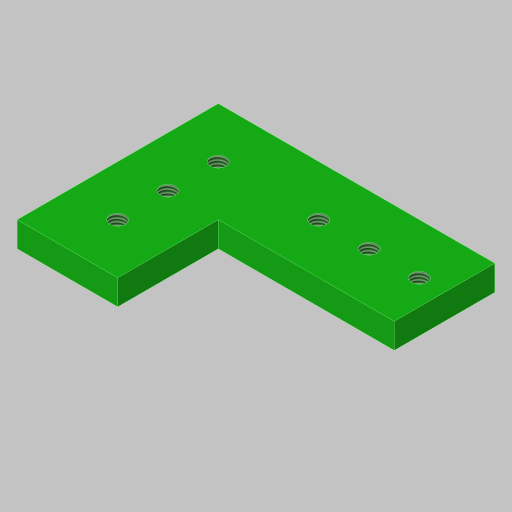
# Autodesk Inventor part: DB1-004
Saved by Autodesk Inventor 2023.5 (Build 275446000, 446)
## iProperties
Created: 2025-01-09
Part Number: DB1-004
Material: Aluminum 6061
Document SubType Name: Modeling
Designer: mavericks
Density: 2.7 g/cm^3
Appearance: Dark Green
Author: mavericks
Autodesk Inventor part; units mm, degrees
ref_plane "YZ Plane" through (0, 0, 0) normal (1, 0, 0) x (0, 1, 0)
ref_plane "XZ Plane" through (0, 0, 0) normal (0, 1, 0) x (-1, 0, 0)
ref_plane "XY Plane" through (0, 0, 0) normal (0, 0, 1) x (1, 0, 0)
sketch "Sketch1" plane through (0, 0, 0) normal (0, 1, 0) x (-1, 0, 0)
  line L0 (12.7, 25.4) -> (-12.7, 25.4)
  line L1 (-12.7, 25.4) -> (-12.7, -25.4)
  line L2 (-12.7, -25.4) -> (12.7, -25.4)
  line L3 (12.7, -25.4) -> (12.7, 25.4)
  line L4 (12.7, 25.4) -> (-12.7, -25.4) construction
  line L5 (-12.7, 25.4) -> (12.7, -25.4) construction
  point P0 (0, 0)
  dimension "d0" = 25.4
  dimension "d1" = 50.8
  constraints: 12 end point, 2 midpoint, 2 parallel, 1 horizontal, 1 perpendicular
  measures "d0" distance of L2.end L1.end
  measures "d1" distance of L1.end L0.end
extrude "Extrusion1" add sketch "Sketch1" along normal blind 6.35
sketch "Sketch3" plane through (12.7, 0, 25.4) normal (1, 0, 0) x (0, 0, -1)
  line L0 (0, 6.35) -> (50.8, 6.35) projected
  line L1 (50.8, 6.35) -> (25.4, 6.35)
  line L2 (25.4, 6.35) -> (25.4, 0)
  line L3 (25.4, 0) -> (50.8, 0)
  line L4 (50.8, 0) -> (50.8, 6.35)
  dimension "d14" = 25.4
  constraints: 8 end point, 2 parallel, 1 horizontal, 1 perpendicular
  measures "d14" distance of L3.end L2.end
extrude "Extrusion2" add sketch "Sketch3" along normal blind 44.45
sketch "Sketch4" plane through (0, 6.35, 0) normal (0, 1, 0) x (1, 0, 0)
  line L0 (-12.7, -25.4) -> (12.7, -25.4) projected
  point P0 (0, 0)
  point P1 (0, -12.7)
  point P2 (0, 0)
  point P3 (0, 12.7)
  point P4 (0, -25.4)
  point P5 (0, -25.4)
  point P6 (0, -25.4)
  point P7 (25.4, 12.7)
  point P8 (38.1, 12.7)
  point P9 (50.8, 12.7)
  dimension "d17" = 12.7
  dimension "d18" = 12.7
  dimension "d19" = 12.7
  dimension "d20" = 25.4
  dimension "d21" = 12.7
  dimension "d22" = 12.7
  constraints: 3 horizontal alignment, 3 midpoint, 3 vertical alignment
  measures "d17" distance from line of L0 point (0, -12.7)
  measures "d18" distance of point (0, -12.7) point (0, 0)
  measures "d19" distance of point (0, 0) point (0, 12.7)
  measures "d20" distance of point (25.4, 12.7) point (0, 12.7)
  measures "d21" distance of point (38.1, 12.7) point (25.4, 12.7)
  measures "d22" distance of point (50.8, 12.7) point (38.1, 12.7)
hole "Hole2" at (0, 6.35, 12.7) at (0, 6.35, 0) at (0, 6.35, -12.7) at (25.4, 6.35, -12.7) at (38.1, 6.35, -12.7) at (50.8, 6.35, -12.7) direction (0, -1, 0) diameter 3.9624 end through all thread size "10-32 UNF" class "2B" standard "ANSI Unified Screw Threads"
body "Solid1"
